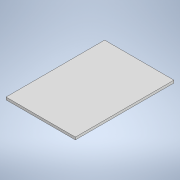
# Autodesk Inventor part: pcb_connecteur
Saved by Autodesk Inventor 2021 (Build 250183000, 183)
## iProperties
Created: 2021-01-15
Part Number: pcb_connecteur
Material: Générique
Document SubType Name: Modeling
Designer: dimercur
Density: 1 g/cm^3
Appearance: Par défaut
Author: dimercur
Autodesk Inventor part; units mm, degrees
ref_plane "YZ Plane" through (0, 0, 0) normal (1, 0, 0) x (0, 1, 0)
ref_plane "XZ Plane" through (0, 0, 0) normal (0, 1, 0) x (-1, 0, 0)
ref_plane "XY Plane" through (0, 0, 0) normal (0, 0, 1) x (1, 0, 0)
sketch "Esquisse1" plane through (0, 0, 0) normal (0, 1, 0) x (-1, 0, 0)
  line L0 (22.5, 32) -> (-22.5, 32)
  line L1 (-22.5, 32) -> (-22.5, -32)
  line L2 (-22.5, -32) -> (22.5, -32)
  line L3 (22.5, -32) -> (22.5, 32)
  point P0 (0, 0)
  dimension "d0" = 64
  dimension "d1" = 45
  dimension "d2" = 22.5
  dimension "d3" = 32
  constraints: 8 end point, 2 parallel, 1 horizontal, 1 perpendicular
  measures "d0" distance of L2.end L0.start
  measures "d1" distance of L0.start L0.end
  measures "d2" horizontal distance of point (0, 0) L0.start
  measures "d3" vertical distance of point (0, 0) L0.start
extrude "Extrusion1" add sketch "Esquisse1" along normal blind 1.6
equation "\"d2\" = 0.5 * d1"
equation "\"d3\" = 0.5 * d0"
